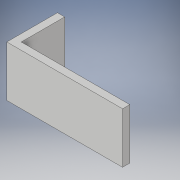
# Autodesk Inventor part: AluminumBracket2-ver1-1111-2019
Saved by Autodesk Inventor 2018 (Build 220112000, 112)
## iProperties
Created: 2020-01-14
Part Number: AluminumBracket2-ver1-1111-2019
Material: Generic
Document SubType Name: Modeling
Designer: Power Hawks CADD
Density: 1 g/cm^3
Appearance: Default
Author: Power Hawks CADD
Autodesk Inventor part; units mm, degrees
ref_plane "YZ Plane" through (0, 0, 0) normal (1, 0, 0) x (0, 1, 0)
ref_plane "XZ Plane" through (0, 0, 0) normal (0, 1, 0) x (-1, 0, 0)
ref_plane "XY Plane" through (0, 0, 0) normal (0, 0, 1) x (1, 0, 0)
sketch "Sketch1" plane through (0, 0, 0) normal (0, 1, 0) x (-1, 0, 0)
  line L0 (0, 0) -> (3.175, 0)
  line L1 (3.175, 0) -> (3.175, -22.225)
  line L2 (3.175, -22.225) -> (0, -22.225)
  line L3 (0, -22.225) -> (0, 0)
  line L4 (3.175, 0) -> (-47.625, 0)
  line L5 (-47.625, 0) -> (-47.625, -3.175)
  line L6 (-47.625, -3.175) -> (3.175, -3.175)
  line L7 (3.175, -3.175) -> (3.175, 0)
  dimension "d0" = 3.175
  dimension "d1" = 22.225
  dimension "d2" = 3.175
  dimension "d3" = 50.8
  constraints: 16 end point, 4 parallel, 2 horizontal, 2 perpendicular
  measures "d0" distance between parallel lines of L1 L3
  measures "d1" distance between parallel lines of L2 L0
  measures "d2" distance between parallel lines of L6 L4
  measures "d3" distance between parallel lines of L5 L1
extrude "Extrusion1" add sketch "Sketch1" along normal blind 22.225
body "Solid1"
